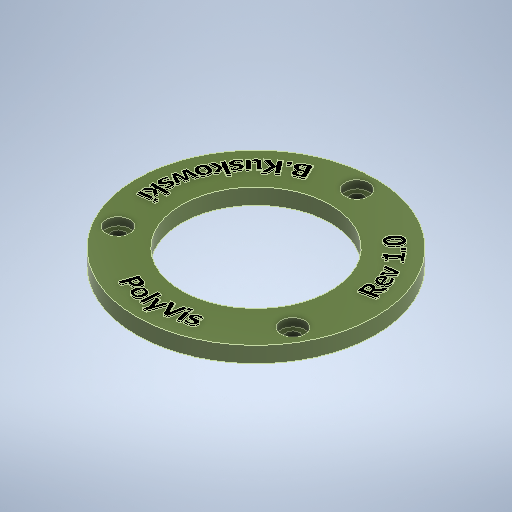
# Autodesk Inventor part: name_plate
Saved by Autodesk Inventor 2025 (Build 290162000, 162)
## iProperties
Created: 2026-08-15
Part Number: name_plate
Material: Ogólny
Document SubType Name: Modeling
Designer: zzapa
Density: 1 g/cm^3
Appearance: Ciemnooliwkowa
Author: zzapa
Autodesk Inventor part; units mm, degrees
(part 1 of 2)
ref_plane "YZ Plane" through (0, 0, 0) normal (1, 0, 0) x (0, 1, 0)
ref_plane "XZ Plane" through (0, 0, 0) normal (0, 1, 0) x (-1, 0, 0)
ref_plane "XY Plane" through (0, 0, 0) normal (0, 0, 1) x (1, 0, 0)
sketch "Szkic1" plane through (0, 0, 0) normal (0, 1, 0) x (-1, 0, 0)
  circle A0 centre (0, 0) radius 14
  circle A1 centre (0, 0) radius 22.5
  dimension "d13" = 28
  dimension "d14" = 45
  constraints: 2 centre point, 2 coincident
  measures "d13" diameter of A0
  measures "d14" diameter of A1
extrude "Wyciągnięcie proste1" add sketch "Szkic1" along normal blind 3
sketch "Szkic2" plane through (0, 3, 0) normal (0, 1, 0) x (1, 0, 0)
  line L0 (0, 31.5) -> (0, -31.5) projected
  point P0 (0, 0)
  point P1 (0, 19)
  point P2 (-16.454483, -9.5)
  point P3 (16.454483, -9.5)
  dimension "d4" = 360
  dimension "d15" = 19
  constraints: 1 point on line, 4 other
  measures "d15" distance of point (0, 0) point (0, 19)
hole "Otwór1" at (0, 3, -19) at (-16.454483, 3, 9.5) at (16.454483, 3, 9.5) direction (0, -1, 0) diameter 2.6 end through all counterbore diameter 4.5 counterbore depth 1.5
sketch "Szkic3" plane through (0, 3, 0) normal (0, 1, 0) x (1, 0, 0)
  circle A0 centre (0, 0) radius 14
  circle A1 centre (0, 0) radius 22.5
  circle A2 centre (0, 0) radius 14
  line L0 (0, -14) -> (0, -22.5)
  line L1 (0, 31.5) -> (0, -31.5)
  circle A3 centre (0, 0) radius 20
  spline S0 degree 2 poles (-9.49756, 16.58394) (-9.596722, 16.78857) (-9.590845, 17.173188) (-9.51142, 17.338018) knots 0 0 0 1 2 2 2
  spline S1 degree 2 poles (-9.51142, 17.338018) (-9.415005, 17.5358) (-9.095361, 17.817037) (-8.808434, 17.956079) knots 0 0 0 1 2 2 2
  line L2 (-8.808434, 17.956079) -> (-7.711884, 18.487455)
  line L3 (-7.711884, 18.487455) -> (-6.381826, 15.742743)
  line L4 (-6.381826, 15.742743) -> (-7.349371, 15.273881)
  spline S2 degree 2 poles (-7.349371, 15.273881) (-7.651868, 15.127295) (-7.985896, 15.023106) (-8.157143, 15.030757) knots 0 0 0 1 2 2 2
  spline S3 degree 2 poles (-8.157143, 15.030757) (-8.343892, 15.03639) (-8.617809, 15.233239) (-8.70188, 15.40673) knots 0 0 0 1 2 2 2
  spline S4 degree 2 poles (-8.70188, 15.40673) (-8.798886, 15.606912) (-8.75068, 16.017536) (-8.60831, 16.177163) knots 0 0 0 1 2 2 2
  line L5 (-8.60831, 16.177163) -> (-8.614777, 16.190508)
  spline S5 degree 2 poles (-8.614777, 16.190508) (-8.896433, 16.119938) (-9.361752, 16.303686) (-9.49756, 16.58394) knots 0 0 0 1 2 2 2
  spline S6 degree 2 poles (-8.780414, 16.917728) (-8.7179, 16.788722) (-8.545525, 16.693727) (-8.424886, 16.705496) knots 0 0 0 1 2 2 2
  spline S7 degree 2 poles (-8.424886, 16.705496) (-8.350751, 16.711209) (-8.128396, 16.813467) (-7.946008, 16.90185) knots 0 0 0 1 2 2 2
  line L6 (-7.946008, 16.90185) -> (-7.819226, 16.963287)
  line L7 (-7.819226, 16.963287) -> (-8.154435, 17.655026)
  line L8 (-8.154435, 17.655026) -> (-8.192248, 17.636702)
  spline S8 degree 2 poles (-8.192248, 17.636702) (-8.459156, 17.507361) (-8.660553, 17.401527) (-8.744682, 17.303082) knots 0 0 0 1 2 2 2
  spline S9 degree 2 poles (-8.744682, 17.303082) (-8.817621, 17.215552) (-8.828917, 17.017819) (-8.780414, 16.917728) knots 0 0 0 1 2 2 2
  spline S10 degree 2 poles (-8.066993, 15.881929) (-8.034658, 15.815202) (-7.897802, 15.708488) (-7.811537, 15.71184) knots 0 0 0 1 2 2 2
  spline S11 degree 2 poles (-7.811537, 15.71184) (-7.72972, 15.713035) (-7.540728, 15.799126) (-7.356116, 15.888587) knots 0 0 0 1 2 2 2
  line L9 (-7.356116, 15.888587) -> (-7.309407, 15.911221)
  line L10 (-7.309407, 15.911221) -> (-7.591802, 16.493972)
  line L11 (-7.591802, 16.493972) -> (-7.678547, 16.451936)
  spline S12 degree 2 poles (-7.678547, 16.451936) (-7.854262, 16.366787) (-7.99338, 16.291132) (-8.051759, 16.218898) knots 0 0 0 1 2 2 2
  spline S13 degree 2 poles (-8.051759, 16.218898) (-8.114654, 16.138981) (-8.111185, 15.973123) (-8.066993, 15.881929) knots 0 0 0 1 2 2 2
  line L12 (-10.858692, 16.799376) -> (-10.243501, 17.181464)
  line L13 (-10.243501, 17.181464) -> (-9.81838, 16.496985)
  line L14 (-9.81838, 16.496985) -> (-10.43357, 16.114897)
  line L15 (-10.43357, 16.114897) -> (-10.858692, 16.799376)
  line L16 (-13.490215, 14.844099) -> (-12.758811, 15.413419)
  line L17 (-12.758811, 15.413419) -> (-11.344812, 14.944855)
  line L18 (-11.344812, 14.944855) -> (-11.353365, 15.201299)
  line L19 (-11.353365, 15.201299) -> (-11.986448, 16.01462)
  line L20 (-11.986448, 16.01462) -> (-11.381821, 16.485258)
  line L21 (-11.381821, 16.485258) -> (-9.50838, 14.078451)
  line L22 (-9.50838, 14.078451) -> (-10.113007, 13.607814)
  line L23 (-10.113007, 13.607814) -> (-10.949528, 14.68249)
  line L24 (-10.949528, 14.68249) -> (-10.88537, 13.006612)
  line L25 (-10.88537, 13.006612) -> (-11.581666, 12.46462)
  line L26 (-11.581666, 12.46462) -> (-11.593406, 14.250207)
  line L27 (-11.593406, 14.250207) -> (-13.490215, 14.844099)
  line L28 (-15.108638, 13.147971) -> (-14.609945, 13.662822)
  line L29 (-14.609945, 13.662822) -> (-14.427084, 13.4857)
  spline S14 degree 2 poles (-14.427084, 13.4857) (-14.409958, 13.727188) (-14.310458, 14.064377) (-14.16085, 14.218832) knots 0 0 0 1 2 2 2
  spline S15 degree 2 poles (-14.16085, 14.218832) (-13.923541, 14.46383) (-13.346312, 14.438073) (-13.033851, 14.135418) knots 0 0 0 1 2 2 2
  line L30 (-13.033851, 14.135418) -> (-11.957991, 13.093321)
  line L31 (-11.957991, 13.093321) -> (-12.460123, 12.57492)
  line L32 (-12.460123, 12.57492) -> (-13.280333, 13.36939)
  spline S16 degree 2 poles (-13.280333, 13.36939) (-13.408158, 13.493203) (-13.583528, 13.638982) (-13.662638, 13.667436) knots 0 0 0 1 2 2 2
  spline S17 degree 2 poles (-13.662638, 13.667436) (-13.738198, 13.69245) (-13.886038, 13.646395) (-13.97202, 13.557628) knots 0 0 0 1 2 2 2
  spline S18 degree 2 poles (-13.97202, 13.557628) (-14.023609, 13.504367) (-14.114798, 13.303649) (-14.128826, 13.196802) knots 0 0 0 1 2 2 2
  line L33 (-14.128826, 13.196802) -> (-12.957097, 12.061845)
  line L34 (-12.957097, 12.061845) -> (-13.45579, 11.546994)
  line L35 (-13.45579, 11.546994) -> (-15.108638, 13.147971)
  spline S19 degree 2 poles (-15.924854, 12.201865) (-15.772571, 12.402782) (-15.410718, 12.696068) (-15.262046, 12.769466) knots 0 0 0 1 2 2 2
  line L36 (-15.262046, 12.769466) -> (-14.77945, 12.403688)
  line L37 (-14.77945, 12.403688) -> (-14.815281, 12.356413)
  spline S20 degree 2 poles (-14.815281, 12.356413) (-14.87815, 12.338935) (-15.032129, 12.29127) (-15.143664, 12.230043) knots 0 0 0 1 2 2 2
  spline S21 degree 2 poles (-15.143664, 12.230043) (-15.242302, 12.177648) (-15.446276, 12.019011) (-15.535854, 11.900824) knots 0 0 0 1 2 2 2
  spline S22 degree 2 poles (-15.535854, 11.900824) (-15.626925, 11.780668) (-15.692413, 11.538776) (-15.611652, 11.477564) knots 0 0 0 1 2 2 2
  spline S23 degree 2 poles (-15.611652, 11.477564) (-15.548619, 11.429789) (-15.417449, 11.463728) (-15.297308, 11.564953) knots 0 0 0 1 2 2 2
  spline S24 degree 2 poles (-15.297308, 11.564953) (-15.230312, 11.616519) (-15.042096, 11.7871) (-14.960233, 11.846006) knots 0 0 0 1 2 2 2
  spline S25 degree 2 poles (-14.960233, 11.846006) (-14.729034, 12.01192) (-14.302826, 12.030031) (-14.08812, 11.867297) knots 0 0 0 1 2 2 2
  spline S26 degree 2 poles (-14.08812, 11.867297) (-13.965994, 11.774733) (-13.834418, 11.498229) (-13.833324, 11.323723) knots 0 0 0 1 2 2 2
  spline S27 degree 2 poles (-13.833324, 11.323723) (-13.832706, 11.152681) (-13.977572, 10.756958) (-14.131348, 10.554071) knots 0 0 0 1 2 2 2
  spline S28 degree 2 poles (-14.131348, 10.554071) (-14.277659, 10.361033) (-14.599327, 10.096215) (-14.736118, 10.026218) knots 0 0 0 1 2 2 2
  line L38 (-14.736118, 10.026218) -> (-15.200986, 10.378559)
  line L39 (-15.200986, 10.378559) -> (-15.166647, 10.423864)
  spline S29 degree 2 poles (-15.166647, 10.423864) (-15.120615, 10.435495) (-14.946751, 10.505304) (-14.874385, 10.543496) knots 0 0 0 1 2 2 2
  spline S30 degree 2 poles (-14.874385, 10.543496) (-14.787628, 10.59249) (-14.609926, 10.736925) (-14.539756, 10.829505) knots 0 0 0 1 2 2 2
  spline S31 degree 2 poles (-14.539756, 10.829505) (-14.445699, 10.953601) (-14.400511, 11.189169) (-14.469453, 11.241423) knots 0 0 0 1 2 2 2
  spline S32 degree 2 poles (-14.469453, 11.241423) (-14.532486, 11.289198) (-14.667596, 11.258245) (-14.810546, 11.143294) knots 0 0 0 1 2 2 2
  spline S33 degree 2 poles (-14.810546, 11.143294) (-14.883514, 11.083849) (-15.061818, 10.918161) (-15.158549, 10.851916) knots 0 0 0 1 2 2 2
  spline S34 degree 2 poles (-15.158549, 10.851916) (-15.370879, 10.702713) (-15.77237, 10.684477) (-15.977227, 10.839746) knots 0 0 0 1 2 2 2
  spline S35 degree 2 poles (-15.977227, 10.839746) (-16.105263, 10.936789) (-16.248595, 11.234609) (-16.242287, 11.406605) knots 0 0 0 1 2 2 2
  spline S36 degree 2 poles (-16.242287, 11.406605) (-16.240872, 11.588513) (-16.09356, 11.97928) (-15.924854, 12.201865) knots 0 0 0 1 2 2 2
  line L40 (-17.906375, 9.004858) -> (-17.474165, 9.73992)
  line L41 (-17.474165, 9.73992) -> (-16.297695, 9.77071)
  line L42 (-16.297695, 9.77071) -> (-16.369156, 9.941755)
  line L43 (-16.369156, 9.941755) -> (-17.102088, 10.372713)
  line L44 (-17.102088, 10.372713) -> (-16.738781, 10.990591)
  line L45 (-16.738781, 10.990591) -> (-13.992418, 9.375753)
  line L46 (-13.992418, 9.375753) -> (-14.355725, 8.757875)
  line L47 (-14.355725, 8.757875) -> (-15.894029, 9.662384)
  line L48 (-15.894029, 9.662384) -> (-15.463001, 8.620452)
  line L49 (-15.463001, 8.620452) -> (-15.892706, 7.889651)
  line L50 (-15.892706, 7.889651) -> (-16.338675, 9.086598)
  line L51 (-16.338675, 9.086598) -> (-17.906375, 9.004858)
  spline S37 degree 2 poles (-17.801187, 6.314796) (-18.323942, 6.538164) (-18.68021, 7.365036) (-18.457813, 7.885518) knots 0 0 0 1 2 2 2
  spline S38 degree 2 poles (-18.457813, 7.885518) (-18.236387, 8.403726) (-17.39065, 8.722368) (-16.867896, 8.499) knots 0 0 0 1 2 2 2
  spline S39 degree 2 poles (-16.867896, 8.499) (-16.340596, 8.273689) (-15.988543, 7.443242) (-16.209969, 6.925034) knots 0 0 0 1 2 2 2
  spline S40 degree 2 poles (-16.209969, 6.925034) (-16.431395, 6.406825) (-17.27616, 6.090456) (-17.801187, 6.314796) knots 0 0 0 1 2 2 2
  spline S41 degree 2 poles (-17.517296, 6.991773) (-17.32865, 6.911166) (-17.050143, 6.864733) (-16.951831, 6.887233) knots 0 0 0 1 2 2 2
  spline S42 degree 2 poles (-16.951831, 6.887233) (-16.847031, 6.912336) (-16.722539, 7.03385) (-16.682721, 7.127036) knots 0 0 0 1 2 2 2
  spline S43 degree 2 poles (-16.682721, 7.127036) (-16.643874, 7.21795) (-16.637239, 7.384447) (-16.689265, 7.476561) knots 0 0 0 1 2 2 2
  spline S44 degree 2 poles (-16.689265, 7.476561) (-16.737717, 7.564459) (-16.965414, 7.742387) (-17.160878, 7.825907) knots 0 0 0 1 2 2 2
  spline S45 degree 2 poles (-17.160878, 7.825907) (-17.35407, 7.908456) (-17.619912, 7.946789) (-17.714979, 7.925591) knots 0 0 0 1 2 2 2
  spline S46 degree 2 poles (-17.714979, 7.925591) (-17.810047, 7.904393) (-17.946214, 7.774429) (-17.987003, 7.678969) knots 0 0 0 1 2 2 2
  spline S47 degree 2 poles (-17.987003, 7.678969) (-18.020994, 7.59942) (-18.022733, 7.40664) (-17.975913, 7.327502) knots 0 0 0 1 2 2 2
  spline S48 degree 2 poles (-17.975913, 7.327502) (-17.920643, 7.23669) (-17.717307, 7.077236) (-17.517296, 6.991773) knots 0 0 0 1 2 2 2
  line L52 (-17.612856, 2.532) -> (-19.680749, 3.744774)
  line L53 (-19.680749, 3.744774) -> (-19.495236, 4.483088)
  line L54 (-19.495236, 4.483088) -> (-17.953388, 4.513622)
  line L55 (-17.953388, 4.513622) -> (-19.297677, 5.269345)
  line L56 (-19.297677, 5.269345) -> (-19.112163, 6.007659)
  line L57 (-19.112163, 6.007659) -> (-16.717815, 6.094127)
  line L58 (-16.717815, 6.094127) -> (-16.901522, 5.363004)
  line L59 (-16.901522, 5.363004) -> (-18.464281, 5.391241)
  line L60 (-18.464281, 5.391241) -> (-17.09366, 4.598321)
  line L61 (-17.09366, 4.598321) -> (-17.248455, 3.98226)
  line L62 (-17.248455, 3.98226) -> (-18.825068, 3.955364)
  line L63 (-18.825068, 3.955364) -> (-17.433366, 3.246343)
  line L64 (-17.433366, 3.246343) -> (-17.612856, 2.532)
  spline S49 degree 2 poles (-19.952667, 2.092264) (-19.927688, 2.343131) (-19.772197, 2.782194) (-19.683719, 2.922416) knots 0 0 0 1 2 2 2
  line L65 (-19.683719, 2.922416) -> (-19.081147, 2.862418)
  line L66 (-19.081147, 2.862418) -> (-19.087025, 2.80339)
  spline S50 degree 2 poles (-19.087025, 2.80339) (-19.131519, 2.75566) (-19.237958, 2.634613) (-19.301117, 2.524161) knots 0 0 0 1 2 2 2
  spline S51 degree 2 poles (-19.301117, 2.524161) (-19.357888, 2.427975) (-19.449028, 2.18618) (-19.463721, 2.038612) knots 0 0 0 1 2 2 2
  spline S52 degree 2 poles (-19.463721, 2.038612) (-19.47866, 1.888584) (-19.408219, 1.648087) (-19.307381, 1.638047) knots 0 0 0 1 2 2 2
  spline S53 degree 2 poles (-19.307381, 1.638047) (-19.228678, 1.63021) (-19.134525, 1.727641) (-19.084909, 1.8767) knots 0 0 0 1 2 2 2
  spline S54 degree 2 poles (-19.084909, 1.8767) (-19.054693, 1.955659) (-18.983229, 2.199413) (-18.944164, 2.292394) knots 0 0 0 1 2 2 2
  spline S55 degree 2 poles (-18.944164, 2.292394) (-18.833604, 2.55461) (-18.479556, 2.792581) (-18.211473, 2.765888) knots 0 0 0 1 2 2 2
  spline S56 degree 2 poles (-18.211473, 2.765888) (-18.058985, 2.750705) (-17.802402, 2.583577) (-17.710358, 2.435316) knots 0 0 0 1 2 2 2
  spline S57 degree 2 poles (-17.710358, 2.435316) (-17.620529, 2.289759) (-17.537473, 1.87662) (-17.562697, 1.623294) knots 0 0 0 1 2 2 2
  spline S58 degree 2 poles (-17.562697, 1.623294) (-17.586696, 1.382266) (-17.722778, 0.988463) (-17.802898, 0.857344) knots 0 0 0 1 2 2 2
  line L67 (-17.802898, 0.857344) -> (-18.383334, 0.915138)
  line L68 (-18.383334, 0.915138) -> (-18.377701, 0.971706)
  spline S59 degree 2 poles (-18.377701, 0.971706) (-18.344514, 1.00566) (-18.232677, 1.155975) (-18.190897, 1.226331) knots 0 0 0 1 2 2 2
  spline S60 degree 2 poles (-18.190897, 1.226331) (-18.142485, 1.313413) (-18.066336, 1.529378) (-18.054826, 1.644973) knots 0 0 0 1 2 2 2
  spline S61 degree 2 poles (-18.054826, 1.644973) (-18.039398, 1.79992) (-18.12385, 2.024425) (-18.209932, 2.032996) knots 0 0 0 1 2 2 2
  spline S62 degree 2 poles (-18.209932, 2.032996) (-18.288635, 2.040833) (-18.387706, 1.943891) (-18.449609, 1.771217) knots 0 0 0 1 2 2 2
  spline S63 degree 2 poles (-18.449609, 1.771217) (-18.480805, 1.682421) (-18.546371, 1.448015) (-18.594283, 1.341012) knots 0 0 0 1 2 2 2
  spline S64 degree 2 poles (-18.594283, 1.341012) (-18.697475, 1.102901) (-19.030378, 0.877727) (-19.286164, 0.903196) knots 0 0 0 1 2 2 2
  spline S65 degree 2 poles (-19.286164, 0.903196) (-19.44603, 0.919114) (-19.723769, 1.098284) (-19.808189, 1.248269) knots 0 0 0 1 2 2 2
  spline S66 degree 2 poles (-19.808189, 1.248269) (-19.901957, 1.404154) (-19.98034, 1.814343) (-19.952667, 2.092264) knots 0 0 0 1 2 2 2
  line L69 (-19.97349, -1.668965) -> (-19.988647, -0.816385)
  line L70 (-19.988647, -0.816385) -> (-19.001334, -0.175882)
  line L71 (-19.001334, -0.175882) -> (-19.151586, -0.067312)
  line L72 (-19.151586, -0.067312) -> (-20.001695, -0.082425)
  line L73 (-20.001695, -0.082425) -> (-20.014435, 0.634236)
  line L74 (-20.014435, 0.634236) -> (-16.828999, 0.690866)
  line L75 (-16.828999, 0.690866) -> (-16.816258, -0.025795)
  line L76 (-16.816258, -0.025795) -> (-18.600498, -0.057515)
  line L77 (-18.600498, -0.057515) -> (-17.688883, -0.721116)
  line L78 (-17.688883, -0.721116) -> (-17.673814, -1.568754)
  line L79 (-17.673814, -1.568754) -> (-18.679106, -0.780745)
  line L80 (-18.679106, -0.780745) -> (-19.97349, -1.668965)
  line L81 (-19.833258, -2.601981) -> (-19.913747, -1.88974)
  line L82 (-19.913747, -1.88974) -> (-17.627207, -1.631343)
  line L83 (-17.627207, -1.631343) -> (-17.546718, -2.343584)
  line L84 (-17.546718, -2.343584) -> (-19.833258, -2.601981)
  line L85 (-17.217572, -2.328774) -> (-17.302779, -1.574781)
  line L86 (-17.302779, -1.574781) -> (-16.747722, -1.512055)
  line L87 (-16.747722, -1.512055) -> (-16.662515, -2.266049)
  line L88 (-16.662515, -2.266049) -> (-17.217572, -2.328774)
  spline S67 degree 2 poles (-4.32012, -17.430029) (-4.385879, -17.632162) (-4.634433, -17.956768) (-4.794064, -18.039992) knots 0 0 0 1 2 2 2
  spline S68 degree 2 poles (-4.794064, -18.039992) (-4.892159, -18.093851) (-5.112078, -18.16266) (-5.232374, -18.172908) knots 0 0 0 1 2 2 2
  spline S69 degree 2 poles (-5.232374, -18.172908) (-5.35502, -18.182393) (-5.623333, -18.152286) (-5.778459, -18.10182) knots 0 0 0 1 2 2 2
  line L89 (-5.778459, -18.10182) -> (-6.159222, -17.977949)
  line L90 (-6.159222, -17.977949) -> (-6.468134, -18.927506)
  line L91 (-6.468134, -18.927506) -> (-7.196754, -18.69047)
  line L92 (-7.196754, -18.69047) -> (-6.253197, -15.79009)
  line L93 (-6.253197, -15.79009) -> (-5.127361, -16.15635)
  spline S70 degree 2 poles (-5.127361, -16.15635) (-4.878219, -16.237401) (-4.54373, -16.447584) (-4.42777, -16.594472) knots 0 0 0 1 2 2 2
  spline S71 degree 2 poles (-4.42777, -16.594472) (-4.299181, -16.758465) (-4.238305, -17.178537) (-4.32012, -17.430029) knots 0 0 0 1 2 2 2
  spline S72 degree 2 poles (-5.073661, -17.205678) (-5.033135, -17.081108) (-5.093307, -16.866597) (-5.162516, -16.807694) knots 0 0 0 1 2 2 2
  spline S73 degree 2 poles (-5.162516, -16.807694) (-5.251405, -16.729393) (-5.434848, -16.65412) (-5.597025, -16.60136) knots 0 0 0 1 2 2 2
  line L94 (-5.597025, -16.60136) -> (-5.700442, -16.567716)
  line L95 (-5.700442, -16.567716) -> (-5.983356, -17.43736)
  line L96 (-5.983356, -17.43736) -> (-5.931648, -17.454182)
  spline S74 degree 2 poles (-5.931648, -17.454182) (-5.830581, -17.487061) (-5.645721, -17.542002) (-5.573737, -17.552424) knots 0 0 0 1 2 2 2
  spline S75 degree 2 poles (-5.573737, -17.552424) (-5.511919, -17.562138) (-5.364296, -17.547784) (-5.317571, -17.523997) knots 0 0 0 1 2 2 2
  spline S76 degree 2 poles (-5.317571, -17.523997) (-5.219419, -17.477954) (-5.11648, -17.3373) (-5.073661, -17.205678) knots 0 0 0 1 2 2 2
  spline S77 degree 2 poles (-2.227592, -18.756246) (-2.329998, -19.315422) (-3.057775, -19.845504) (-3.61452, -19.743543) knots 0 0 0 1 2 2 2
  spline S78 degree 2 poles (-3.61452, -19.743543) (-4.168834, -19.642027) (-4.666384, -18.887543) (-4.563978, -18.328366) knots 0 0 0 1 2 2 2
  spline S79 degree 2 poles (-4.563978, -18.328366) (-4.460682, -17.764327) (-3.728488, -17.237568) (-3.174174, -17.339083) knots 0 0 0 1 2 2 2
  spline S80 degree 2 poles (-3.174174, -17.339083) (-2.61986, -17.440599) (-2.124741, -18.194638) (-2.227592, -18.756246) knots 0 0 0 1 2 2 2
  spline S81 degree 2 poles (-2.95055, -18.628871) (-2.913595, -18.427081) (-2.929815, -18.145196) (-2.973471, -18.05428) knots 0 0 0 1 2 2 2
  spline S82 degree 2 poles (-2.973471, -18.05428) (-3.021099, -17.957612) (-3.167105, -17.863028) (-3.266785, -17.844773) knots 0 0 0 1 2 2 2
  spline S83 degree 2 poles (-3.266785, -17.844773) (-3.364033, -17.826964) (-3.527885, -17.857262) (-3.606234, -17.928347) knots 0 0 0 1 2 2 2
  spline S84 degree 2 poles (-3.606234, -17.928347) (-3.681262, -17.995014) (-3.804511, -18.256383) (-3.842802, -18.465466) knots 0 0 0 1 2 2 2
  spline S85 degree 2 poles (-3.842802, -18.465466) (-3.880647, -18.672118) (-3.859324, -18.939862) (-3.817654, -19.027901) knots 0 0 0 1 2 2 2
  spline S86 degree 2 poles (-3.817654, -19.027901) (-3.775984, -19.11594) (-3.619158, -19.220043) (-3.517047, -19.238743) knots 0 0 0 1 2 2 2
  spline S87 degree 2 poles (-3.517047, -19.238743) (-3.431955, -19.254327) (-3.243551, -19.213448) (-3.176707, -19.150307) knots 0 0 0 1 2 2 2
  spline S88 degree 2 poles (-3.176707, -19.150307) (-3.100344, -19.076346) (-2.989732, -18.842816) (-2.95055, -18.628871) knots 0 0 0 1 2 2 2
  line L97 (-1.338835, -19.958356) -> (-2.053028, -19.897576)
  line L98 (-2.053028, -19.897576) -> (-1.782871, -16.72311)
  line L99 (-1.782871, -16.72311) -> (-1.068678, -16.78389)
  line L100 (-1.068678, -16.78389) -> (-1.338835, -19.958356)
  line L101 (1.336045, -17.68966) -> (0.199736, -20.841927)
  line L102 (0.199736, -20.841927) -> (-0.571394, -20.847534)
  line L103 (-0.571394, -20.847534) -> (-0.229443, -19.945348)
  line L104 (-0.229443, -19.945348) -> (-1.088567, -17.707289)
  line L105 (-1.088567, -17.707289) -> (-0.337209, -17.701826)
  line L106 (-0.337209, -17.701826) -> (0.157714, -19.141701)
  line L107 (0.157714, -19.141701) -> (0.599517, -17.695015)
  line L108 (0.599517, -17.695015) -> (1.336045, -17.68966)
  line L109 (3.767167, -16.586537) -> (3.155195, -19.752961)
  line L110 (3.155195, -19.752961) -> (2.364672, -19.864399)
  line L111 (2.364672, -19.864399) -> (0.901216, -16.990543)
  line L112 (0.901216, -16.990543) -> (1.686844, -16.879795)
  line L113 (1.686844, -16.879795) -> (2.633978, -18.835494)
  line L114 (2.633978, -18.835494) -> (3.001118, -16.694525)
  line L115 (3.001118, -16.694525) -> (3.767167, -16.586537)
  line L116 (5.177609, -19.321511) -> (4.482049, -19.494606)
  line L117 (4.482049, -19.494606) -> (3.926354, -17.261618)
  line L118 (3.926354, -17.261618) -> (4.621915, -17.088523)
  line L119 (4.621915, -17.088523) -> (5.177609, -19.321511)
  line L120 (4.564116, -16.764153) -> (3.827782, -16.947395)
  line L121 (3.827782, -16.947395) -> (3.692887, -16.405337)
  line L122 (3.692887, -16.405337) -> (4.429221, -16.222095)
  line L123 (4.429221, -16.222095) -> (4.564116, -16.764153)
  spline S89 degree 2 poles (6.390481, -19.017051) (6.15193, -19.098607) (5.687961, -19.139683) (5.52365, -19.117495) knots 0 0 0 1 2 2 2
  line L124 (5.52365, -19.117495) -> (5.327757, -18.544504)
  line L125 (5.327757, -18.544504) -> (5.383887, -18.525314)
  spline S90 degree 2 poles (5.383887, -18.525314) (5.445793, -18.545943) (5.60013, -18.592439) (5.726841, -18.603973) knots 0 0 0 1 2 2 2
  spline S91 degree 2 poles (5.726841, -18.603973) (5.837921, -18.615627) (6.095722, -18.598017) (6.236046, -18.550044) knots 0 0 0 1 2 2 2
  spline S92 degree 2 poles (6.236046, -18.550044) (6.378709, -18.50127) (6.568167, -18.33724) (6.535385, -18.241351) knots 0 0 0 1 2 2 2
  spline S93 degree 2 poles (6.535385, -18.241351) (6.509799, -18.166512) (6.382048, -18.121376) (6.225853, -18.138206) knots 0 0 0 1 2 2 2
  spline S94 degree 2 poles (6.225853, -18.138206) (6.141478, -18.143543) (5.890074, -18.179863) (5.789269, -18.182981) knots 0 0 0 1 2 2 2
  spline S95 degree 2 poles (5.789269, -18.182981) (5.504822, -18.191415) (5.14122, -17.968315) (5.054068, -17.713393) knots 0 0 0 1 2 2 2
  spline S96 degree 2 poles (5.054068, -17.713393) (5.004495, -17.568391) (5.049851, -17.265555) (5.146439, -17.120214) knots 0 0 0 1 2 2 2
  spline S97 degree 2 poles (5.146439, -17.120214) (5.241488, -16.978011) (5.582725, -16.730746) (5.823614, -16.648391) knots 0 0 0 1 2 2 2
  spline S98 degree 2 poles (5.823614, -16.648391) (6.052811, -16.570034) (6.467547, -16.530117) (6.620104, -16.548487) knots 0 0 0 1 2 2 2
  line L126 (6.620104, -16.548487) -> (6.8088, -17.100429)
  line L127 (6.8088, -17.100429) -> (6.755009, -17.118819)
  spline S99 degree 2 poles (6.755009, -17.118819) (6.710334, -17.102748) (6.527133, -17.063508) (6.445777, -17.054753) knots 0 0 0 1 2 2 2
  spline S100 degree 2 poles (6.445777, -17.054753) (6.346451, -17.046917) (6.118374, -17.067425) (6.008453, -17.105004) knots 0 0 0 1 2 2 2
  spline S101 degree 2 poles (6.008453, -17.105004) (5.861113, -17.155377) (5.692024, -17.325504) (5.720008, -17.40736) knots 0 0 0 1 2 2 2
  spline S102 degree 2 poles (5.720008, -17.40736) (5.745594, -17.4822) (5.874944, -17.532013) (6.057725, -17.516542) knots 0 0 0 1 2 2 2
  spline S103 degree 2 poles (6.057725, -17.516542) (6.151455, -17.508007) (6.391905, -17.470208) (6.509141, -17.469309) knots 0 0 0 1 2 2 2
  spline S104 degree 2 poles (6.509141, -17.469309) (6.768601, -17.464192) (7.111775, -17.67338) (7.194929, -17.916609) knots 0 0 0 1 2 2 2
  spline S105 degree 2 poles (7.194929, -17.916609) (7.246901, -18.068627) (7.199385, -18.39571) (7.09806, -18.534834) knots 0 0 0 1 2 2 2
  spline S106 degree 2 poles (7.09806, -18.534834) (6.995255, -18.684913) (6.654758, -18.926701) (6.390481, -19.017051) knots 0 0 0 1 2 2 2
  line L128 (19.259047, 5.629037) -> (19.447781, 4.716544)
  line L129 (19.447781, 4.716544) -> (18.523051, 3.659563)
  line L130 (18.523051, 3.659563) -> (18.57912, 3.388478)
  line L131 (18.57912, 3.388478) -> (19.675564, 3.615259)
  line L132 (19.675564, 3.615259) -> (19.829756, 2.869774)
  line L133 (19.829756, 2.869774) -> (16.842974, 2.252007)
  line L134 (16.842974, 2.252007) -> (16.594666, 3.452528)
  spline S107 degree 2 poles (16.594666, 3.452528) (16.543102, 3.70183) (16.529938, 4.082748) (16.594214, 4.260099) knots 0 0 0 1 2 2 2
  spline S108 degree 2 poles (16.594214, 4.260099) (16.66283, 4.440872) (16.940855, 4.695246) (17.182895, 4.745308) knots 0 0 0 1 2 2 2
  spline S109 degree 2 poles (17.182895, 4.745308) (17.524173, 4.815895) (18.016664, 4.594693) (18.196092, 4.361742) knots 0 0 0 1 2 2 2
  line L135 (18.196092, 4.361742) -> (19.259047, 5.629037)
  spline S110 degree 2 poles (17.436489, 3.995143) (17.32273, 3.971614) (17.178585, 3.850937) (17.155543, 3.742689) knots 0 0 0 1 2 2 2
  spline S111 degree 2 poles (17.155543, 3.742689) (17.141016, 3.66649) (17.159617, 3.491137) (17.18615, 3.362855) knots 0 0 0 1 2 2 2
  line L136 (17.18615, 3.362855) -> (17.238215, 3.111133)
  line L137 (17.238215, 3.111133) -> (18.04179, 3.27734)
  line L138 (18.04179, 3.27734) -> (17.997235, 3.492756)
  spline S112 degree 2 poles (17.997235, 3.492756) (17.965195, 3.647662) (17.880912, 3.859909) (17.804882, 3.922426) knots 0 0 0 1 2 2 2
  spline S113 degree 2 poles (17.804882, 3.922426) (17.731774, 3.983023) (17.56235, 4.021175) (17.436489, 3.995143) knots 0 0 0 1 2 2 2
  spline S114 degree 2 poles (18.829313, 6.926439) (19.048234, 6.311747) (18.694503, 5.448503) (18.151991, 5.255288) knots 0 0 0 1 2 2 2
  spline S115 degree 2 poles (18.151991, 5.255288) (17.621121, 5.066219) (16.77054, 5.450697) (16.574837, 6.000194) knots 0 0 0 1 2 2 2
  spline S116 degree 2 poles (16.574837, 6.000194) (16.398207, 6.496138) (16.756944, 7.190624) (17.255216, 7.368083) knots 0 0 0 1 2 2 2
  line L139 (17.255216, 7.368083) -> (17.499696, 7.455155)
  line L140 (17.499696, 7.455155) -> (18.027928, 5.971979)
  spline S117 degree 2 poles (18.027928, 5.971979) (18.175955, 6.035194) (18.337221, 6.215943) (18.366247, 6.325982) knots 0 0 0 1 2 2 2
  spline S118 degree 2 poles (18.366247, 6.325982) (18.396102, 6.433692) (18.364402, 6.684773) (18.315476, 6.822147) knots 0 0 0 1 2 2 2
  spline S119 degree 2 poles (18.315476, 6.822147) (18.274014, 6.938566) (18.141523, 7.148504) (18.063284, 7.228211) knots 0 0 0 1 2 2 2
  spline S120 degree 2 poles (18.063284, 7.228211) (17.998506, 7.299594) (17.862601, 7.408614) (17.814248, 7.441244) knots 0 0 0 1 2 2 2
  line L141 (17.814248, 7.441244) -> (17.788541, 7.513424)
  line L142 (17.788541, 7.513424) -> (18.347351, 7.712444)
  spline S121 degree 2 poles (18.347351, 7.712444) (18.409802, 7.640232) (18.513779, 7.525088) (18.584841, 7.413963) knots 0 0 0 1 2 2 2
  spline S122 degree 2 poles (18.584841, 7.413963) (18.654084, 7.31531) (18.769607, 7.094082) (18.829313, 6.926439) knots 0 0 0 1 2 2 2
  spline S123 degree 2 poles (17.329395, 6.64412) (17.116843, 6.563173) (16.95816, 6.294137) (17.026988, 6.100882) knots 0 0 0 1 2 2 2
  spline S124 degree 2 poles (17.026988, 6.100882) (17.097474, 5.90297) (17.414576, 5.764029) (17.621291, 5.824532) knots 0 0 0 1 2 2 2
  line L143 (17.621291, 5.824532) -> (17.329395, 6.64412)
  line L144 (15.275905, 9.020575) -> (17.702871, 9.314447)
  line L145 (17.702871, 9.314447) -> (18.054181, 8.614113)
  line L146 (18.054181, 8.614113) -> (16.364188, 6.851086)
  line L147 (16.364188, 6.851086) -> (16.026178, 7.524909)
  line L148 (16.026178, 7.524909) -> (17.173198, 8.628439)
  line L149 (17.173198, 8.628439) -> (15.607266, 8.360007)
  line L150 (15.607266, 8.360007) -> (15.275905, 9.020575)
  line L151 (15.221292, 13.018303) -> (16.446221, 11.41915)
  line L152 (16.446221, 11.41915) -> (16.024359, 11.096009)
  line L153 (16.024359, 11.096009) -> (15.633584, 11.606169)
  line L154 (15.633584, 11.606169) -> (14.352299, 10.624722)
  line L155 (14.352299, 10.624722) -> (14.743074, 10.114563)
  line L156 (14.743074, 10.114563) -> (14.348682, 9.812464)
  spline S125 degree 2 poles (14.348682, 9.812464) (14.263012, 9.924306) (14.063743, 10.123485) (13.981247, 10.16615) knots 0 0 0 1 2 2 2
  spline S126 degree 2 poles (13.981247, 10.16615) (13.883388, 10.212614) (13.685792, 10.198249) (13.581673, 10.130949) knots 0 0 0 1 2 2 2
  line L157 (13.581673, 10.130949) -> (13.175868, 10.66073)
  line L158 (13.175868, 10.66073) -> (15.181187, 12.196776)
  line L159 (15.181187, 12.196776) -> (14.79943, 12.695163)
  line L160 (14.79943, 12.695163) -> (15.221292, 13.018303)
  line L161 (14.344815, 13.94118) -> (14.840085, 13.412826)
  line L162 (14.840085, 13.412826) -> (14.252223, 12.861775)
  line L163 (14.252223, 12.861775) -> (13.756953, 13.390129)
  line L164 (13.756953, 13.390129) -> (14.344815, 13.94118)
  spline S127 degree 2 poles (11.273228, 14.684046) (11.533476, 14.981806) (12.018758, 15.345493) (12.256586, 15.40352) knots 0 0 0 1 2 2 2
  spline S128 degree 2 poles (12.256586, 15.40352) (12.490926, 15.461314) (12.961144, 15.319511) (13.203075, 15.108059) knots 0 0 0 1 2 2 2
  spline S129 degree 2 poles (13.203075, 15.108059) (13.446866, 14.894981) (13.648469, 14.4496) (13.621169, 14.204285) knots 0 0 0 1 2 2 2
  spline S130 degree 2 poles (13.621169, 14.204285) (13.595496, 13.96083) (13.303288, 13.434958) (13.04304, 13.137198) knots 0 0 0 1 2 2 2
  spline S131 degree 2 poles (13.04304, 13.137198) (12.776286, 12.831993) (12.304016, 12.483195) (12.059448, 12.421211) knots 0 0 0 1 2 2 2
  spline S132 degree 2 poles (12.059448, 12.421211) (11.818133, 12.362948) (11.347445, 12.511727) (11.112959, 12.716672) knots 0 0 0 1 2 2 2
  spline S133 degree 2 poles (11.112959, 12.716672) (10.865446, 12.933003) (10.670818, 13.378853) (10.699744, 13.626029) knots 0 0 0 1 2 2 2
  spline S134 degree 2 poles (10.699744, 13.626029) (10.727278, 13.867857) (11.021113, 14.395591) (11.273228, 14.684046) knots 0 0 0 1 2 2 2
  spline S135 degree 2 poles (11.851999, 14.178189) (11.47952, 13.75202) (11.318183, 13.285743) (11.483812, 13.14098) knots 0 0 0 1 2 2 2
  spline S136 degree 2 poles (11.483812, 13.14098) (11.649441, 12.996218) (12.091789, 13.216885) (12.465895, 13.644916) knots 0 0 0 1 2 2 2
  spline S137 degree 2 poles (12.465895, 13.644916) (12.833495, 14.065502) (12.997851, 14.538988) (12.832221, 14.683751) knots 0 0 0 1 2 2 2
  spline S138 degree 2 poles (12.832221, 14.683751) (12.668453, 14.826887) (12.221226, 14.600637) (11.851999, 14.178189) knots 0 0 0 1 2 2 2
  point P0 (0, -18.25)
  dimension "d16" = 40
  constraints: 2 end point, 2 vertical alignment, 1 centre point, 1 coincident, 1 collinear, 1 midpoint, 1 vertical, 5 other
  measures "d16" diameter of A3
sketch "Szkic3 outline for Wyciągnięcie proste2" plane through (0, 3, 0) normal (0, 1, 0) x (1, 0, 0)
  spline S0 degree 2 poles (-9.49756, 16.58394) (-9.596722, 16.78857) (-9.590845, 17.173188) (-9.51142, 17.338018) knots 0 0 0 0.5 1 1 1
  spline S1 degree 2 poles (-8.614777, 16.190508) (-8.896433, 16.119938) (-9.361752, 16.303686) (-9.49756, 16.58394) knots 0 0 0 0.5 1 1 1
  spline S2 degree 2 poles (-9.51142, 17.338018) (-9.415005, 17.5358) (-9.095361, 17.817037) (-8.808434, 17.956079) knots 0 0 0 0.5 1 1 1
  line L0 (-8.60831, 16.177163) -> (-8.614777, 16.190508)
  line L1 (-8.808434, 17.956079) -> (-7.711884, 18.487455)
  spline S3 degree 2 poles (-8.70188, 15.40673) (-8.798886, 15.606912) (-8.75068, 16.017536) (-8.60831, 16.177163) knots 0 0 0 0.5 1 1 1
  line L2 (-7.711884, 18.487455) -> (-6.381826, 15.742743)
  spline S4 degree 2 poles (-8.157143, 15.030757) (-8.343892, 15.03639) (-8.617809, 15.233239) (-8.70188, 15.40673) knots 0 0 0 0.5 1 1 1
  line L3 (-6.381826, 15.742743) -> (-7.349371, 15.273881)
  spline S5 degree 2 poles (-7.349371, 15.273881) (-7.651868, 15.127295) (-7.985896, 15.023106) (-8.157143, 15.030757) knots 0 0 0 0.5 1 1 1
  spline S6 degree 2 poles (-8.051759, 16.218898) (-8.114654, 16.138981) (-8.111185, 15.973123) (-8.066993, 15.881929) knots 0 0 0 0.5 1 1 1
  spline S7 degree 2 poles (-8.066993, 15.881929) (-8.034658, 15.815202) (-7.897802, 15.708488) (-7.811537, 15.71184) knots 0 0 0 0.5 1 1 1
  spline S8 degree 2 poles (-7.811537, 15.71184) (-7.72972, 15.713035) (-7.540728, 15.799126) (-7.356116, 15.888587) knots 0 0 0 0.5 1 1 1
  line L4 (-7.356116, 15.888587) -> (-7.309407, 15.911221)
  line L5 (-7.309407, 15.911221) -> (-7.591802, 16.493972)
  line L6 (-7.591802, 16.493972) -> (-7.678547, 16.451936)
  spline S9 degree 2 poles (-7.678547, 16.451936) (-7.854262, 16.366787) (-7.99338, 16.291132) (-8.051759, 16.218898) knots 0 0 0 0.5 1 1 1
  spline S10 degree 2 poles (-8.744682, 17.303082) (-8.817621, 17.215552) (-8.828917, 17.017819) (-8.780414, 16.917728) knots 0 0 0 0.5 1 1 1
  spline S11 degree 2 poles (-8.780414, 16.917728) (-8.7179, 16.788722) (-8.545525, 16.693727) (-8.424886, 16.705496) knots 0 0 0 0.5 1 1 1
  spline S12 degree 2 poles (-8.424886, 16.705496) (-8.350751, 16.711209) (-8.128396, 16.813467) (-7.946008, 16.90185) knots 0 0 0 0.5 1 1 1
  line L7 (-7.946008, 16.90185) -> (-7.819226, 16.963287)
  line L8 (-7.819226, 16.963287) -> (-8.154435, 17.655026)
  line L9 (-8.154435, 17.655026) -> (-8.192248, 17.636702)
  spline S13 degree 2 poles (-8.192248, 17.636702) (-8.459156, 17.507361) (-8.660553, 17.401527) (-8.744682, 17.303082) knots 0 0 0 0.5 1 1 1
  line L10 (-10.858692, 16.799376) -> (-10.243501, 17.181464)
  line L11 (-10.243501, 17.181464) -> (-9.81838, 16.496985)
  line L12 (-9.81838, 16.496985) -> (-10.43357, 16.114897)
  line L13 (-10.43357, 16.114897) -> (-10.858692, 16.799376)
  line L14 (-13.490215, 14.844099) -> (-12.758811, 15.413419)
  line L15 (-12.758811, 15.413419) -> (-11.344812, 14.944855)
  line L16 (-11.344812, 14.944855) -> (-11.353365, 15.201299)
  line L17 (-11.353365, 15.201299) -> (-11.986448, 16.01462)
  line L18 (-11.986448, 16.01462) -> (-11.381821, 16.485258)
  line L19 (-11.381821, 16.485258) -> (-9.50838, 14.078451)
  line L20 (-9.50838, 14.078451) -> (-10.113007, 13.607814)
  line L21 (-10.113007, 13.607814) -> (-10.949528, 14.68249)
  line L22 (-10.949528, 14.68249) -> (-10.88537, 13.006612)
  line L23 (-10.88537, 13.006612) -> (-11.581666, 12.46462)
  line L24 (-11.581666, 12.46462) -> (-11.593406, 14.250207)
  line L25 (-11.593406, 14.250207) -> (-13.490215, 14.844099)
  line L26 (-15.108638, 13.147971) -> (-14.609945, 13.662822)
  line L27 (-14.609945, 13.662822) -> (-14.427084, 13.4857)
  spline S14 degree 2 poles (-14.427084, 13.4857) (-14.409958, 13.727188) (-14.310458, 14.064377) (-14.16085, 14.218832) knots 0 0 0 0.5 1 1 1
  spline S15 degree 2 poles (-14.16085, 14.218832) (-13.923541, 14.46383) (-13.346312, 14.438073) (-13.033851, 14.135418) knots 0 0 0 0.5 1 1 1
  line L28 (-13.033851, 14.135418) -> (-11.957991, 13.093321)
  line L29 (-11.957991, 13.093321) -> (-12.460123, 12.57492)
  line L30 (-12.460123, 12.57492) -> (-13.280333, 13.36939)
  spline S16 degree 2 poles (-13.280333, 13.36939) (-13.408158, 13.493203) (-13.583528, 13.638982) (-13.662638, 13.667436) knots 0 0 0 0.5 1 1 1
  spline S17 degree 2 poles (-13.662638, 13.667436) (-13.738198, 13.69245) (-13.886038, 13.646395) (-13.97202, 13.557628) knots 0 0 0 0.5 1 1 1
  spline S18 degree 2 poles (-13.97202, 13.557628) (-14.023609, 13.504367) (-14.114798, 13.303649) (-14.128826, 13.196802) knots 0 0 0 0.5 1 1 1
  line L31 (-14.128826, 13.196802) -> (-12.957097, 12.061845)
  line L32 (-12.957097, 12.061845) -> (-13.45579, 11.546994)
  line L33 (-13.45579, 11.546994) -> (-15.108638, 13.147971)
  spline S19 degree 2 poles (-15.924854, 12.201865) (-15.772571, 12.402782) (-15.410718, 12.696068) (-15.262046, 12.769466) knots 0 0 0 0.5 1 1 1
  line L34 (-15.262046, 12.769466) -> (-14.77945, 12.403688)
  line L35 (-14.77945, 12.403688) -> (-14.815281, 12.356413)
  spline S20 degree 2 poles (-14.815281, 12.356413) (-14.87815, 12.338935) (-15.032129, 12.29127) (-15.143664, 12.230043) knots 0 0 0 0.5 1 1 1
  spline S21 degree 2 poles (-15.143664, 12.230043) (-15.242302, 12.177648) (-15.446276, 12.019011) (-15.535854, 11.900824) knots 0 0 0 0.5 1 1 1
  spline S22 degree 2 poles (-15.535854, 11.900824) (-15.626925, 11.780668) (-15.692413, 11.538776) (-15.611652, 11.477564) knots 0 0 0 0.5 1 1 1
  spline S23 degree 2 poles (-15.611652, 11.477564) (-15.548619, 11.429789) (-15.417449, 11.463728) (-15.297308, 11.564953) knots 0 0 0 0.5 1 1 1
  spline S24 degree 2 poles (-15.297308, 11.564953) (-15.230312, 11.616519) (-15.042096, 11.7871) (-14.960233, 11.846006) knots 0 0 0 0.5 1 1 1
  spline S25 degree 2 poles (-14.960233, 11.846006) (-14.729034, 12.01192) (-14.302826, 12.030031) (-14.08812, 11.867297) knots 0 0 0 0.5 1 1 1
  spline S26 degree 2 poles (-14.08812, 11.867297) (-13.965994, 11.774733) (-13.834418, 11.498229) (-13.833324, 11.323723) knots 0 0 0 0.5 1 1 1
  spline S27 degree 2 poles (-13.833324, 11.323723) (-13.832706, 11.152681) (-13.977572, 10.756958) (-14.131348, 10.554071) knots 0 0 0 0.5 1 1 1
  spline S28 degree 2 poles (-14.131348, 10.554071) (-14.277659, 10.361033) (-14.599327, 10.096215) (-14.736118, 10.026218) knots 0 0 0 0.5 1 1 1
  line L36 (-14.736118, 10.026218) -> (-15.200986, 10.378559)
  line L37 (-15.200986, 10.378559) -> (-15.166647, 10.423864)
  spline S29 degree 2 poles (-15.166647, 10.423864) (-15.120615, 10.435495) (-14.946751, 10.505304) (-14.874385, 10.543496) knots 0 0 0 0.5 1 1 1
  spline S30 degree 2 poles (-14.874385, 10.543496) (-14.787628, 10.59249) (-14.609926, 10.736925) (-14.539756, 10.829505) knots 0 0 0 0.5 1 1 1
  spline S31 degree 2 poles (-14.539756, 10.829505) (-14.445699, 10.953601) (-14.400511, 11.189169) (-14.469453, 11.241423) knots 0 0 0 0.5 1 1 1
  spline S32 degree 2 poles (-14.469453, 11.241423) (-14.532486, 11.289198) (-14.667596, 11.258245) (-14.810546, 11.143294) knots 0 0 0 0.5 1 1 1
  spline S33 degree 2 poles (-14.810546, 11.143294) (-14.883514, 11.083849) (-15.061818, 10.918161) (-15.158549, 10.851916) knots 0 0 0 0.5 1 1 1
  spline S34 degree 2 poles (-15.158549, 10.851916) (-15.370879, 10.702713) (-15.77237, 10.684477) (-15.977227, 10.839746) knots 0 0 0 0.5 1 1 1
  spline S35 degree 2 poles (-15.977227, 10.839746) (-16.105263, 10.936789) (-16.248595, 11.234609) (-16.242287, 11.406605) knots 0 0 0 0.5 1 1 1
  spline S36 degree 2 poles (-16.242287, 11.406605) (-16.240872, 11.588513) (-16.09356, 11.97928) (-15.924854, 12.201865) knots 0 0 0 0.5 1 1 1
  line L38 (-17.906375, 9.004858) -> (-17.474165, 9.73992)
  line L39 (-17.474165, 9.73992) -> (-16.297695, 9.77071)
  line L40 (-16.297695, 9.77071) -> (-16.369156, 9.941755)
  line L41 (-16.369156, 9.941755) -> (-17.102088, 10.372713)
  line L42 (-17.102088, 10.372713) -> (-16.738781, 10.990591)
  line L43 (-16.738781, 10.990591) -> (-13.992418, 9.375753)
  line L44 (-13.992418, 9.375753) -> (-14.355725, 8.757875)
  line L45 (-14.355725, 8.757875) -> (-15.894029, 9.662384)
  line L46 (-15.894029, 9.662384) -> (-15.463001, 8.620452)
  line L47 (-15.463001, 8.620452) -> (-15.892706, 7.889651)
  line L48 (-15.892706, 7.889651) -> (-16.338675, 9.086598)
  line L49 (-16.338675, 9.086598) -> (-17.906375, 9.004858)
  spline S37 degree 2 poles (-17.801187, 6.314796) (-18.323942, 6.538164) (-18.68021, 7.365036) (-18.457813, 7.885518) knots 0 0 0 0.5 1 1 1
  spline S38 degree 2 poles (-16.209969, 6.925034) (-16.431395, 6.406825) (-17.27616, 6.090456) (-17.801187, 6.314796) knots 0 0 0 0.5 1 1 1
  spline S39 degree 2 poles (-18.457813, 7.885518) (-18.236387, 8.403726) (-17.39065, 8.722368) (-16.867896, 8.499) knots 0 0 0 0.5 1 1 1
  spline S40 degree 2 poles (-16.867896, 8.499) (-16.340596, 8.273689) (-15.988543, 7.443242) (-16.209969, 6.925034) knots 0 0 0 0.5 1 1 1
  spline S41 degree 2 poles (-17.975913, 7.327502) (-17.920643, 7.23669) (-17.717307, 7.077236) (-17.517296, 6.991773) knots 0 0 0 0.5 1 1 1
  spline S42 degree 2 poles (-17.517296, 6.991773) (-17.32865, 6.911166) (-17.050143, 6.864733) (-16.951831, 6.887233) knots 0 0 0 0.5 1 1 1
  spline S43 degree 2 poles (-16.951831, 6.887233) (-16.847031, 6.912336) (-16.722539, 7.03385) (-16.682721, 7.127036) knots 0 0 0 0.5 1 1 1
  spline S44 degree 2 poles (-16.682721, 7.127036) (-16.643874, 7.21795) (-16.637239, 7.384447) (-16.689265, 7.476561) knots 0 0 0 0.5 1 1 1
  spline S45 degree 2 poles (-16.689265, 7.476561) (-16.737717, 7.564459) (-16.965414, 7.742387) (-17.160878, 7.825907) knots 0 0 0 0.5 1 1 1
  spline S46 degree 2 poles (-17.160878, 7.825907) (-17.35407, 7.908456) (-17.619912, 7.946789) (-17.714979, 7.925591) knots 0 0 0 0.5 1 1 1
  spline S47 degree 2 poles (-17.714979, 7.925591) (-17.810047, 7.904393) (-17.946214, 7.774429) (-17.987003, 7.678969) knots 0 0 0 0.5 1 1 1
  spline S48 degree 2 poles (-17.987003, 7.678969) (-18.020994, 7.59942) (-18.022733, 7.40664) (-17.975913, 7.327502) knots 0 0 0 0.5 1 1 1
  line L50 (-17.612856, 2.532) -> (-19.680749, 3.744774)
  line L51 (-19.680749, 3.744774) -> (-19.495236, 4.483088)
  line L52 (-19.495236, 4.483088) -> (-17.953388, 4.513622)
  line L53 (-17.953388, 4.513622) -> (-19.297677, 5.269345)
  line L54 (-19.297677, 5.269345) -> (-19.112163, 6.007659)
  line L55 (-19.112163, 6.007659) -> (-16.717815, 6.094127)
  line L56 (-16.717815, 6.094127) -> (-16.901522, 5.363004)
  line L57 (-16.901522, 5.363004) -> (-18.464281, 5.391241)
  line L58 (-18.464281, 5.391241) -> (-17.09366, 4.598321)
  line L59 (-17.09366, 4.598321) -> (-17.248455, 3.98226)
  line L60 (-17.248455, 3.98226) -> (-18.825068, 3.955364)
  line L61 (-18.825068, 3.955364) -> (-17.433366, 3.246343)
  line L62 (-17.433366, 3.246343) -> (-17.612856, 2.532)
  spline S49 degree 2 poles (-19.952667, 2.092264) (-19.927688, 2.343131) (-19.772197, 2.782194) (-19.683719, 2.922416) knots 0 0 0 0.5 1 1 1
  line L63 (-19.683719, 2.922416) -> (-19.081147, 2.862418)
  line L64 (-19.081147, 2.862418) -> (-19.087025, 2.80339)
  spline S50 degree 2 poles (-19.087025, 2.80339) (-19.131519, 2.75566) (-19.237958, 2.634613) (-19.301117, 2.524161) knots 0 0 0 0.5 1 1 1
  spline S51 degree 2 poles (-19.301117, 2.524161) (-19.357888, 2.427975) (-19.449028, 2.18618) (-19.463721, 2.038612) knots 0 0 0 0.5 1 1 1
  spline S52 degree 2 poles (-19.463721, 2.038612) (-19.47866, 1.888584) (-19.408219, 1.648087) (-19.307381, 1.638047) knots 0 0 0 0.5 1 1 1
  spline S53 degree 2 poles (-19.307381, 1.638047) (-19.228678, 1.63021) (-19.134525, 1.727641) (-19.084909, 1.8767) knots 0 0 0 0.5 1 1 1
  spline S54 degree 2 poles (-19.084909, 1.8767) (-19.054693, 1.955659) (-18.983229, 2.199413) (-18.944164, 2.292394) knots 0 0 0 0.5 1 1 1
  spline S55 degree 2 poles (-18.944164, 2.292394) (-18.833604, 2.55461) (-18.479556, 2.792581) (-18.211473, 2.765888) knots 0 0 0 0.5 1 1 1
  spline S56 degree 2 poles (-18.211473, 2.765888) (-18.058985, 2.750705) (-17.802402, 2.583577) (-17.710358, 2.435316) knots 0 0 0 0.5 1 1 1
  spline S57 degree 2 poles (-17.710358, 2.435316) (-17.620529, 2.289759) (-17.537473, 1.87662) (-17.562697, 1.623294) knots 0 0 0 0.5 1 1 1
  spline S58 degree 2 poles (-17.562697, 1.623294) (-17.586696, 1.382266) (-17.722778, 0.988463) (-17.802898, 0.857344) knots 0 0 0 0.5 1 1 1
  line L65 (-17.802898, 0.857344) -> (-18.383334, 0.915138)
  line L66 (-18.383334, 0.915138) -> (-18.377701, 0.971706)
  spline S59 degree 2 poles (-18.377701, 0.971706) (-18.344514, 1.00566) (-18.232677, 1.155975) (-18.190897, 1.226331) knots 0 0 0 0.5 1 1 1
  spline S60 degree 2 poles (-18.190897, 1.226331) (-18.142485, 1.313413) (-18.066336, 1.529378) (-18.054826, 1.644973) knots 0 0 0 0.5 1 1 1
  spline S61 degree 2 poles (-18.054826, 1.644973) (-18.039398, 1.79992) (-18.12385, 2.024425) (-18.209932, 2.032996) knots 0 0 0 0.5 1 1 1
  spline S62 degree 2 poles (-18.209932, 2.032996) (-18.288635, 2.040833) (-18.387706, 1.943891) (-18.449609, 1.771217) knots 0 0 0 0.5 1 1 1
  spline S63 degree 2 poles (-18.449609, 1.771217) (-18.480805, 1.682421) (-18.546371, 1.448015) (-18.594283, 1.341012) knots 0 0 0 0.5 1 1 1
  spline S64 degree 2 poles (-18.594283, 1.341012) (-18.697475, 1.102901) (-19.030378, 0.877727) (-19.286164, 0.903196) knots 0 0 0 0.5 1 1 1
  spline S65 degree 2 poles (-19.286164, 0.903196) (-19.44603, 0.919114) (-19.723769, 1.098284) (-19.808189, 1.248269) knots 0 0 0 0.5 1 1 1
  spline S66 degree 2 poles (-19.808189, 1.248269) (-19.901957, 1.404154) (-19.98034, 1.814343) (-19.952667, 2.092264) knots 0 0 0 0.5 1 1 1
  line L67 (-19.97349, -1.668965) -> (-19.988647, -0.816385)
  line L68 (-19.988647, -0.816385) -> (-19.001334, -0.175882)
  line L69 (-19.001334, -0.175882) -> (-19.151586, -0.067312)
  line L70 (-19.151586, -0.067312) -> (-20.001695, -0.082425)
  line L71 (-20.001695, -0.082425) -> (-20.014435, 0.634236)
  line L72 (-20.014435, 0.634236) -> (-16.828999, 0.690866)
  line L73 (-16.828999, 0.690866) -> (-16.816258, -0.025795)
  line L74 (-16.816258, -0.025795) -> (-18.600498, -0.057515)
  line L75 (-18.600498, -0.057515) -> (-17.688883, -0.721116)
  line L76 (-17.688883, -0.721116) -> (-17.673814, -1.568754)
  line L77 (-17.673814, -1.568754) -> (-18.679106, -0.780745)
  line L78 (-18.679106, -0.780745) -> (-19.97349, -1.668965)
  line L79 (-19.833258, -2.601981) -> (-19.913747, -1.88974)
  line L80 (-19.913747, -1.88974) -> (-17.627207, -1.631343)
  line L81 (-17.627207, -1.631343) -> (-17.546718, -2.343584)
  line L82 (-17.546718, -2.343584) -> (-19.833258, -2.601981)
  line L83 (-17.217572, -2.328774) -> (-17.302779, -1.574781)
  line L84 (-17.302779, -1.574781) -> (-16.747722, -1.512055)
  line L85 (-16.747722, -1.512055) -> (-16.662515, -2.266049)
  line L86 (-16.662515, -2.266049) -> (-17.217572, -2.328774)
  spline S67 degree 2 poles (-4.32012, -17.430029) (-4.385879, -17.632162) (-4.634433, -17.956768) (-4.794064, -18.039992) knots 0 0 0 0.5 1 1 1
  spline S68 degree 2 poles (-4.42777, -16.594472) (-4.299181, -16.758465) (-4.238305, -17.178537) (-4.32012, -17.430029) knots 0 0 0 0.5 1 1 1
  spline S69 degree 2 poles (-4.794064, -18.039992) (-4.892159, -18.093851) (-5.112078, -18.16266) (-5.232374, -18.172908) knots 0 0 0 0.5 1 1 1
  spline S70 degree 2 poles (-5.127361, -16.15635) (-4.878219, -16.237401) (-4.54373, -16.447584) (-4.42777, -16.594472) knots 0 0 0 0.5 1 1 1
  spline S71 degree 2 poles (-5.232374, -18.172908) (-5.35502, -18.182393) (-5.623333, -18.152286) (-5.778459, -18.10182) knots 0 0 0 0.5 1 1 1
  line L87 (-6.253197, -15.79009) -> (-5.127361, -16.15635)
  line L88 (-5.778459, -18.10182) -> (-6.159222, -17.977949)
  line L89 (-7.196754, -18.69047) -> (-6.253197, -15.79009)
  line L90 (-6.159222, -17.977949) -> (-6.468134, -18.927506)
  line L91 (-6.468134, -18.927506) -> (-7.196754, -18.69047)
  spline S72 degree 2 poles (-5.317571, -17.523997) (-5.219419, -17.477954) (-5.11648, -17.3373) (-5.073661, -17.205678) knots 0 0 0 0.5 1 1 1
  spline S73 degree 2 poles (-5.073661, -17.205678) (-5.033135, -17.081108) (-5.093307, -16.866597) (-5.162516, -16.807694) knots 0 0 0 0.5 1 1 1
  spline S74 degree 2 poles (-5.162516, -16.807694) (-5.251405, -16.729393) (-5.434848, -16.65412) (-5.597025, -16.60136) knots 0 0 0 0.5 1 1 1
  line L92 (-5.597025, -16.60136) -> (-5.700442, -16.567716)
  line L93 (-5.700442, -16.567716) -> (-5.983356, -17.43736)
  line L94 (-5.983356, -17.43736) -> (-5.931648, -17.454182)
  spline S75 degree 2 poles (-5.931648, -17.454182) (-5.830581, -17.487061) (-5.645721, -17.542002) (-5.573737, -17.552424) knots 0 0 0 0.5 1 1 1
  spline S76 degree 2 poles (-5.573737, -17.552424) (-5.511919, -17.562138) (-5.364296, -17.547784) (-5.317571, -17.523997) knots 0 0 0 0.5 1 1 1
  spline S77 degree 2 poles (-2.227592, -18.756246) (-2.329998, -19.315422) (-3.057775, -19.845504) (-3.61452, -19.743543) knots 0 0 0 0.5 1 1 1
  spline S78 degree 2 poles (-3.174174, -17.339083) (-2.61986, -17.440599) (-2.124741, -18.194638) (-2.227592, -18.756246) knots 0 0 0 0.5 1 1 1
  spline S79 degree 2 poles (-3.61452, -19.743543) (-4.168834, -19.642027) (-4.666384, -18.887543) (-4.563978, -18.328366) knots 0 0 0 0.5 1 1 1
  spline S80 degree 2 poles (-4.563978, -18.328366) (-4.460682, -17.764327) (-3.728488, -17.237568) (-3.174174, -17.339083) knots 0 0 0 0.5 1 1 1
  spline S81 degree 2 poles (-3.176707, -19.150307) (-3.100344, -19.076346) (-2.989732, -18.842816) (-2.95055, -18.628871) knots 0 0 0 0.5 1 1 1
  spline S82 degree 2 poles (-2.95055, -18.628871) (-2.913595, -18.427081) (-2.929815, -18.145196) (-2.973471, -18.05428) knots 0 0 0 0.5 1 1 1
  spline S83 degree 2 poles (-2.973471, -18.05428) (-3.021099, -17.957612) (-3.167105, -17.863028) (-3.266785, -17.844773) knots 0 0 0 0.5 1 1 1
  spline S84 degree 2 poles (-3.266785, -17.844773) (-3.364033, -17.826964) (-3.527885, -17.857262) (-3.606234, -17.928347) knots 0 0 0 0.5 1 1 1
  spline S85 degree 2 poles (-3.606234, -17.928347) (-3.681262, -17.995014) (-3.804511, -18.256383) (-3.842802, -18.465466) knots 0 0 0 0.5 1 1 1
  spline S86 degree 2 poles (-3.842802, -18.465466) (-3.880647, -18.672118) (-3.859324, -18.939862) (-3.817654, -19.027901) knots 0 0 0 0.5 1 1 1
  spline S87 degree 2 poles (-3.817654, -19.027901) (-3.775984, -19.11594) (-3.619158, -19.220043) (-3.517047, -19.238743) knots 0 0 0 0.5 1 1 1
  spline S88 degree 2 poles (-3.517047, -19.238743) (-3.431955, -19.254327) (-3.243551, -19.213448) (-3.176707, -19.150307) knots 0 0 0 0.5 1 1 1
  line L95 (-1.338835, -19.958356) -> (-2.053028, -19.897576)
  line L96 (-2.053028, -19.897576) -> (-1.782871, -16.72311)
  line L97 (-1.782871, -16.72311) -> (-1.068678, -16.78389)